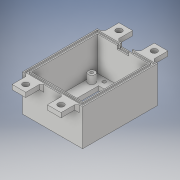
# Autodesk Inventor part: obudowa_baza_V2_cz2
Saved by Autodesk Inventor 2019 (Build 230136000, 136)
## iProperties
Created: 2019-08-14
Part Number: obudowa_baza_V2_cz2
Material: Ogólny
Document SubType Name: Modeling
Designer: mikol
Density: 1 g/cm^3
Appearance: Domyślna
Author: mikol
## iProperties of the stored document obudowa_baza_V2_cz2_3DPrint.ipt
Created: 2019-09-16
Part Number: obudowa_baza_V2_cz2_3DPrint
Material: Ogólny
Document SubType Name: Modeling
Designer: mikol
Density: 1 g/cm^3
Appearance: Domyślna
Author: mikol
Autodesk Inventor part; units mm, degrees
ref_plane "YZ Plane" through (0, 0, 0) normal (1, 0, 0) x (0, 1, 0)
ref_plane "XZ Plane" through (0, 0, 0) normal (0, 1, 0) x (-1, 0, 0)
ref_plane "XY Plane" through (0, 0, 0) normal (0, 0, 1) x (1, 0, 0)
sketch "Sketch2" plane through (0, 0, 0) normal (0, 1, 0) x (-1, 0, 0)
  circle A0 centre (13, 25.5) radius 1.45
  line L0 (26.5, 33) -> (-26.5, 33)
  line L1 (-26.5, 33) -> (-26.5, -33)
  line L2 (-26.5, -33) -> (26.5, -33)
  line L3 (26.5, -33) -> (26.5, 33)
  circle A1 centre (13, -25.5) radius 1.45
  circle A2 centre (-13, 25.5) radius 1.45
  circle A3 centre (-13, -25.5) radius 1.45
  line L4 (37.1, 0) -> (-37.1, 0) projected
  line L5 (0, -46.2) -> (0, 46.2) projected
  circle A4 centre (18.5, 20) radius 1.6
  line L6 (-26.5, 9.9943) -> (-26.5, -14.3434)
  line L7 (26.5, -13.3434) -> (26.5, 10.9943)
  line L8 (10.5, 33) -> (-10.5, 33)
  line L9 (-10.5, 33) -> (-10.5, -33)
  line L10 (-10.5, -33) -> (10.5, -33)
  line L11 (10.5, -33) -> (10.5, 33)
  line L12 (10.5, 33) -> (-10.5, 33)
  line L13 (-10.5, 33) -> (-10.5, 24)
  line L14 (-10.5, 24) -> (10.5, 24)
  line L15 (10.5, 24) -> (10.5, 33)
  line L16 (10.5, -33) -> (-10.5, -33)
  line L17 (-10.5, -33) -> (-10.5, -24)
  line L18 (-10.5, -24) -> (10.5, -24)
  line L19 (10.5, -24) -> (10.5, -33)
  point P0 (0, 0)
  point P1 (26.5, 0)
  point P2 (0, -33)
  dimension "d17" = 2.9
  dimension "d20" = 51
  dimension "d23" = 26
  dimension "d26" = 66
  dimension "d27" = 53
  dimension "d28" = 25.5
  dimension "d29" = 25.5
  dimension "d30" = 13
  dimension "d31" = 13
  dimension "d33" = 3.2
  dimension "d42" = 20
  dimension "d110" = 48
  dimension "d111" = 24
  dimension "d112" = 21
  dimension "d113" = 10.5
  dimension "d163" = 2.9
  dimension "d164" = 2.9
  dimension "d165" = 2.9
  constraints: 36 end point, 9 parallel, 8 point on line, 5 centre point, 5 horizontal, 4 perpendicular, 2 midpoint, 1 vertical, 6 other
  measures "d17" diameter of A0
  measures "d20" distance of A0.centre A1.centre
  measures "d23" distance of A0.centre A2.centre
  measures "d26" distance of L2.end L0.start
  measures "d27" distance of L1.end L2.end
  measures "d28" distance from line of L4 A0.centre
  measures "d29" distance from line of L4 A1.centre
  measures "d30" distance from line of L5 A0.centre
  measures "d31" distance from line of L5 A2.centre
  measures "d33" diameter of A4
  measures "d42" distance from line of L4 A4.centre
  measures "d110" distance between parallel lines of L14 L18
  measures "d111" distance between parallel lines of L4 L18
  measures "d112" distance between parallel lines of L9 L11
  measures "d113" distance between parallel lines of L5 L11
  measures "d163" diameter of A1
  measures "d164" diameter of A3
  measures "d165" diameter of A2
extrude "Extrusion1" add sketch "Sketch2" along normal blind 4 contours L3 L4 L11 L0 | L11 L14 L5 L0 | L5 L14 L9 L0 | L11 L4 L5 L14 | L3 L2 L11 L4 | L9 L4 L1 L0 | L5 L4 L9 L14 | L11 L18 L5 L4 | L5 L18 L9 L4 | L11 L2 L5 L18 | L9 L2 L1 L4 | L5 L2 L9 L18 | A4
sketch "Sketch4" plane through (0, 4, 0) normal (0, 1, 0) x (1, 0, 0)
  circle A0 centre (13, -25.5) radius 1.45 projected
  circle A1 centre (13, 25.5) radius 1.45 projected
  circle A2 centre (-13, 25.5) radius 1.45 projected
  circle A3 centre (-13, -25.5) radius 1.45 projected
  line L0 (26.5, 33) -> (-26.5, 33) projected
  line L1 (-26.5, 33) -> (-26.5, -33) projected
  line L2 (-26.5, -33) -> (26.5, -33) projected
  line L3 (26.5, -33) -> (26.5, 33) projected
  line L4 (-26.5, -33) -> (26.5, -33)
  line L5 (26.5, -33) -> (26.5, 33)
  line L6 (26.5, 33) -> (-26.5, 33)
  line L7 (-26.5, 33) -> (-26.5, -33)
  line L8 (-22.5, -29) -> (22.5, -29)
  line L9 (22.5, -29) -> (22.5, 29)
  line L10 (22.5, 29) -> (-22.5, 29)
  line L11 (-22.5, 29) -> (-22.5, -29)
  point P0 (0, 0)
  dimension "d54" = 4
  dimension "d55" = 4
  dimension "d56" = 4
  dimension "d57" = 4
  constraints: 16 end point, 4 parallel, 2 horizontal, 2 perpendicular
  measures "d54" distance between parallel lines of L1 L11
  measures "d55" distance between parallel lines of L5 L9
  measures "d56" distance between parallel lines of L10 L0
  measures "d57" distance between parallel lines of L2 L8
extrude "Extrusion3" add sketch "Sketch4" along normal blind 30 contours L3 L2 L1 L0
sketch "Sketch5" plane through (0, 4, 0) normal (0, 1, 0) x (1, 0, 0)
  line L0 (-12.5, 20) -> (12.5, 20)
  line L1 (12.5, 20) -> (12.5, -20)
  line L2 (12.5, -20) -> (-12.5, -20)
  line L3 (-12.5, -20) -> (-12.5, 20)
  line L4 (-12.5, 20) -> (12.5, -20) construction
  line L5 (12.5, 20) -> (-12.5, -20) construction
  point P0 (0, 0)
  dimension "d61" = 40
  dimension "d62" = 25
  constraints: 12 end point, 2 midpoint, 2 parallel, 1 horizontal, 1 perpendicular
  measures "d61" distance of L0.end L1.end
  measures "d62" distance of L0.start L0.end
extrude "Extrusion4" cut sketch "Sketch5" against normal blind 15
sketch "Sketch6" plane through (-26.5, 0, 33) normal (0, 0, 1) x (1, 0, 0)
  line L0 (0, 0) -> (53, 0) projected
  line L1 (53, 0) -> (53, 34) projected
  line L2 (0, 34) -> (53, 34) projected
  line L3 (0, 0) -> (0, 34) projected
  line L4 (4, 34) -> (49, 34) projected
  line L5 (5, 34) -> (17, 34)
  line L6 (17, 34) -> (17, 30)
  line L7 (17, 30) -> (5, 30)
  line L8 (5, 30) -> (5, 34)
  point P0 (26.5, 0)
  dimension "d65" = 12
  dimension "d66" = 4
  dimension "d67" = 5
  constraints: 8 end point, 2 parallel, 1 horizontal, 1 perpendicular, 1 point on line
  measures "d65" distance of L6.end L7.end
  measures "d66" distance of L5.end L6.end
  measures "d67" distance between parallel lines of L3 L8
extrude "Extrusion5" add sketch "Sketch6" along normal blind 14 contours L2 L6 L7 L8
chamfer "Chamfer1" distance 2 angle 45 3 edges at (-15.5, 30, 33) (-9.5, 32, 33) (-21.5, 32, 33)
chamfer "Chamfer3" distance 2 angle 45 4 edges at (26.5, 0, 0) (0, 0, 33) (0, 0, -33) (-26.5, 0, 0)
sketch "Sketch10" plane through (26.5, 34, -33) normal (0, 0, -1) x (-1, 0, 0)
  line L0 (53, -32) -> (0, -32) projected
  line L1 (53, -32) -> (53, 0) projected
  line L2 (0, 0) -> (53, 0) projected
  line L3 (0, -32) -> (0, 0) projected
  line L4 (17, 0) -> (5, 0)
  line L5 (5, 0) -> (5, -4)
  line L6 (5, -4) -> (17, -4)
  line L7 (17, -4) -> (17, 0)
  point P0 (26.5, -34)
  dimension "d98" = 12
  dimension "d99" = 4
  dimension "d100" = 5
  constraints: 8 end point, 2 parallel, 1 horizontal, 1 perpendicular, 1 point on line
  measures "d98" distance of L6.end L5.end
  measures "d99" distance of L5.end L4.end
  measures "d100" distance between parallel lines of L3 L5
extrude "Extrusion9" add sketch "Sketch10" along normal blind 14 contours L7 L6 L5 L2
chamfer "Chamfer4" distance 2 angle 45 3 edges at (21.5, 32, -33) (15.5, 30, -33) (9.5, 32, -33)
sketch "Sketch11" plane through (-21.5, 30, 47) normal (0, -1, 0) x (1, 0, 0)
  line L0 (12, -12) -> (0, -12) projected
  line L1 (12, -12) -> (12, 0) projected
  line L2 (0, 0) -> (12, 0) projected
  line L3 (0, -12) -> (0, 0) projected
  line L4 (31, -82) -> (43, -82) projected
  line L5 (31, -82) -> (31, -94) projected
  line L6 (43, -94) -> (31, -94) projected
  line L7 (43, -82) -> (43, -94) projected
  circle A0 centre (6, -6) radius 2.6
  circle A1 centre (37, -88) radius 2.6
  line L8 (0, -12) -> (0, 0) projected
  point P0 (21.5, -47)
  dimension "d106" = 5.2
  dimension "d107" = 5.2
  dimension "d122" = 6
  dimension "d123" = 6
  dimension "d124" = 6
  dimension "d125" = 6
  constraints: 2 centre point
  measures "d106" diameter of A0
  measures "d107" diameter of A1
  measures "d122" distance from line of L5 A1.centre
  measures "d123" distance from line of L6 A1.centre
  measures "d124" distance from line of L2 A0.centre
  measures "d125" distance from line of L8 A0.centre
extrude "Extrusion10" cut sketch "Sketch11" against normal blind 14 contours A0 | A1
mirror "Mirror2" about plane through (0, 0, 0) normal (0, 0, 1)
sketch "Sketch14" plane through (0, 34, 0) normal (0, 1, 0) x (1, 0, 0)
  line L0 (-24.5, -31) -> (24.5, -31) projected
  circle A0 centre (15.5, -41) radius 2.6 projected
  circle A1 centre (-15.5, 41) radius 2.6 projected
  circle A2 centre (15.5, 41) radius 2.6 projected
  line L1 (-22.5, -29) -> (-22.5, 29) projected
  line L2 (-22.5, 29) -> (22.5, 29) projected
  line L3 (22.5, 29) -> (22.5, -29) projected
  line L4 (22.5, -29) -> (-22.5, -29) projected
  line L5 (-21.5, -35) -> (-23.5, -33) projected
  line L6 (-21.5, -35) -> (-21.5, -47) projected
  line L7 (-9.5, -47) -> (-21.5, -47) projected
  line L8 (-9.5, -35) -> (-9.5, -47) projected
  line L9 (-7.5, -33) -> (-9.5, -35) projected
  line L10 (-7.5, -33) -> (7.5, -33) projected
  line L11 (7.5, -33) -> (9.5, -35) projected
  line L12 (9.5, -35) -> (9.5, -47) projected
  line L13 (9.5, -47) -> (21.5, -47) projected
  line L14 (21.5, -35) -> (21.5, -47) projected
  line L15 (21.5, -35) -> (23.5, -33) projected
  line L16 (23.5, -33) -> (26.5, -33) projected
  line L17 (26.5, -33) -> (26.5, 33) projected
  line L18 (26.5, 33) -> (23.5, 33) projected
  line L19 (21.5, 35) -> (23.5, 33) projected
  line L20 (21.5, 35) -> (21.5, 47) projected
  line L21 (9.5, 47) -> (21.5, 47) projected
  line L22 (9.5, 35) -> (9.5, 47) projected
  line L23 (7.5, 33) -> (9.5, 35) projected
  line L24 (7.5, 33) -> (-7.5, 33) projected
  line L25 (-7.5, 33) -> (-9.5, 35) projected
  line L26 (-9.5, 35) -> (-9.5, 47) projected
  line L27 (-9.5, 47) -> (-21.5, 47) projected
  line L28 (-21.5, 35) -> (-21.5, 47) projected
  line L29 (-21.5, 35) -> (-23.5, 33) projected
  line L30 (-23.5, 33) -> (-26.5, 33) projected
  line L31 (-26.5, 33) -> (-26.5, -33) projected
  line L32 (-26.5, -33) -> (-23.5, -33) projected
  circle A3 centre (-15.5, -41) radius 2.6 projected
  line L33 (24.5, -31) -> (26.5, -33) projected
  line L34 (-24.5, 31) -> (-26.5, 33) projected
  line L35 (25.5, -32) -> (-25.5, -32)
  line L36 (-25.5, -32) -> (-25.5, 32)
  line L37 (-25.5, 32) -> (25.5, 32)
  line L38 (25.5, 32) -> (25.5, -32)
  line L39 (23.5, -30) -> (-23.5, -30)
  line L40 (-23.5, -30) -> (-23.5, 30)
  line L41 (-23.5, 30) -> (23.5, 30)
  line L42 (23.5, 30) -> (23.5, -30)
  point P0 (0, 0)
  dimension "d114" = 1
  dimension "d115" = 1
  dimension "d116" = 2
  dimension "d117" = 2
  dimension "d118" = 2
  dimension "d119" = 2
  constraints: 16 end point, 4 parallel, 2 horizontal, 2 midpoint, 2 perpendicular
  measures "d114" distance between parallel lines of L17 L38
  measures "d115" distance between parallel lines of L10 L35
  measures "d116" distance between parallel lines of L36 L40
  measures "d117" distance between parallel lines of L37 L41
  measures "d118" distance between parallel lines of L35 L39
  measures "d119" distance between parallel lines of L38 L42
extrude "Extrusion11" cut sketch "Sketch14" against normal blind 1.2 contours L37 L38 L35 L36
sketch "Sketch15" plane through (26.5, 2, -33) normal (0, 0, -1) x (-1, 0, 0)
  line L0 (50, 32) -> (50, 26) projected
  line L1 (50, 26) -> (34, 26) projected
  line L2 (34, 26) -> (34, 32) projected
  line L3 (19, 32) -> (34, 32) projected
  line L4 (19, 26) -> (19, 32) projected
  line L5 (3, 26) -> (19, 26) projected
  line L6 (3, 32) -> (3, 26) projected
  line L7 (0, 32) -> (3, 32) projected
  line L8 (0, 0) -> (0, 32) projected
  line L9 (53, 0) -> (0, 0) projected
  line L10 (53, 0) -> (53, 32) projected
  line L11 (50, 32) -> (53, 32) projected
  line L12 (52, 32) -> (1, 32) projected
  line L13 (21.5, 32) -> (31.5, 32)
  line L14 (31.5, 32) -> (31.5, 29)
  line L15 (31.5, 29) -> (21.5, 29)
  line L16 (21.5, 29) -> (21.5, 32)
  point P0 (26.5, -2)
  dimension "d126" = 10
  dimension "d127" = 3
  dimension "d128" = 2.5
  dimension "d129" = 2.5
  constraints: 8 end point, 2 parallel, 1 horizontal, 1 perpendicular, 1 point on line
  measures "d126" distance of L14.end L15.end
  measures "d127" distance of L13.end L14.end
  measures "d128" distance between parallel lines of L4 L16
  measures "d129" distance between parallel lines of L2 L14
extrude "Extrusion12" cut sketch "Sketch15" against normal blind 10 contours L14 L15 L16 L3
sketch "Sketch16" plane through (-5, 31, -33) normal (0, 1, 0) x (1, 0, 0)
  line L0 (-21.5, 0) -> (31.5, 0) projected
  line L1 (10, -4) -> (0, -4) projected
  line L2 (10, 0) -> (10, -4) projected
  line L3 (0, 0) -> (10, 0) projected
  line L4 (0, 0) -> (0, -4) projected
  line L5 (0, 0) -> (0, -4) projected
  line L6 (10, -3) -> (0, -3)
  line L7 (0, -3) -> (0, -1)
  line L8 (0, -1) -> (10, -1)
  line L9 (10, -1) -> (10, -3)
  point P0 (5, -33)
  dimension "d132" = 2
  dimension "d133" = 1
  constraints: 8 end point, 2 parallel, 2 point on line, 1 horizontal, 1 perpendicular
  measures "d132" distance of L6.end L7.end
  measures "d133" distance between parallel lines of L1 L6
extrude "Extrusion13" cut sketch "Sketch16" against normal blind 1.2 contours L8 L2 L6 L4
chamfer "Chamfer5" distance 2 angle 45 2 edges at (-5, 32.8, -31) (5, 32.8, -31)
sketch "Sketch17" plane through (0, 4, 0) normal (0, 1, 0) x (1, 0, 0)
  line L0 (-12.5, -20) -> (-12.5, 20) projected
  line L1 (-12.5, 20) -> (12.5, 20) projected
  line L2 (12.5, 20) -> (12.5, -20) projected
  line L3 (12.5, -20) -> (-12.5, -20) projected
  line L4 (-22.5, 29) -> (-22.5, -29) projected
  line L5 (-22.5, -29) -> (22.5, -29) projected
  line L6 (22.5, -29) -> (22.5, 29) projected
  line L7 (22.5, 29) -> (-22.5, 29) projected
  circle A0 centre (13, -25.5) radius 1.45 projected
  circle A1 centre (13, 25.5) radius 1.45 projected
  circle A2 centre (-13, 25.5) radius 1.45 projected
  circle A3 centre (-13, -25.5) radius 1.45 projected
  circle A4 centre (-18.5, -20) radius 1.25
  circle A5 centre (-18.5, 20) radius 1.25
  circle A6 centre (18.5, -20) radius 1.25
  circle A7 centre (18.5, 20) radius 1.25
  circle A8 centre (-18.5, -20) radius 3
  circle A9 centre (-18.5, 20) radius 3
  circle A10 centre (18.5, -20) radius 3
  circle A11 centre (18.5, 20) radius 3
  point P0 (0, 0)
  dimension "d141" = 40
  dimension "d144" = 37
  dimension "d147" = 9
  dimension "d148" = 9
  dimension "d149" = 4
  dimension "d150" = 4
  dimension "d151" = 2.5
  dimension "d154" = 40
  dimension "d157" = 37
  dimension "d160" = 6
  constraints: 8 centre point, 2 horizontal, 2 vertical, 1 coincident, 12 other
  measures "d141" distance of A4.centre A5.centre
  measures "d144" distance of A4.centre A6.centre
  measures "d147" distance from line of L5 A4.centre
  measures "d148" distance from line of L7 A5.centre
  measures "d149" distance from line of L6 A6.centre
  measures "d150" distance from line of L4 A4.centre
  measures "d151" diameter of A4
  measures "d154" distance of A8.centre A9.centre
  measures "d157" distance of A8.centre A10.centre
  measures "d160" diameter of A8
extrude "Extrusion14" add sketch "Sketch17" along normal blind 7 contours A8 | A9 | A10 | A11
equation "\"d28\" = d29"
equation "\"d30\" = d31"
equation "\"d42\" = d43"
equation "\"d55\" = d54"
equation "\"d56\" = d54"
equation "\"d57\" = d54"
equation "\"d128\" = d129"
equation "\"d147\" = d148"
equation "\"d149\" = d150"
equation "\"d43\" = 20"
body "Solid1"
